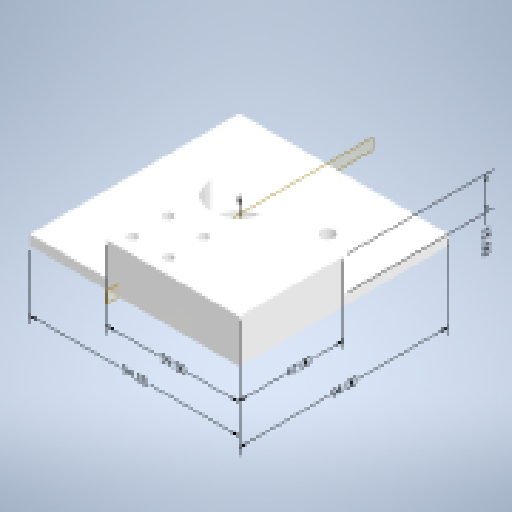
# Autodesk Inventor part: box cover
Saved by Autodesk Inventor 2025.3 (Build 293356000, 356)
## iProperties
Created: 2026-04-05
Part Number: box cover
Material: Wood (Birch)
Document SubType Name: Modeling
Designer: logien
Density: 0.55 g/cm^3
Appearance: Smooth - White
Author: logien
Autodesk Inventor part; units mm, degrees
ref_plane "YZ Plane" through (0, 0, 0) normal (1, 0, 0) x (0, 1, 0)
sketch "Sketch1" plane through (0, 0, 0) normal (0, 1, 0) x (-1, 0, 0)
  line L0 (0, 0) -> (94, 0)
  line L1 (94, 0) -> (94, -94)
  line L2 (94, -94) -> (0, -94)
  line L3 (0, -94) -> (0, 0)
  dimension "d0" = 94
  dimension "d1" = 94
  constraints: 8 end point, 2 parallel, 1 horizontal, 1 perpendicular
  measures "d0" distance of L0.end L1.end
  measures "d1" distance of L0.start L0.end
extrude "Extrusion1" add sketch "Sketch1" along normal blind 4.5
sketch "Sketch2" plane through (0, 4.5, 0) normal (0, 1, 0) x (1, 0, 0)
  circle A0 centre (-47, 47) radius 12.5
  point P0 (0, 0)
  dimension "d4" = 25
  dimension "d5" = 47
  dimension "d6" = 47
  constraints: 1 centre point
  measures "d4" diameter of A0
  measures "d5" horizontal distance of point (0, 0) A0.centre
  measures "d6" horizontal distance of point (0, 0) A0.centre
extrude "Extrusion2" cut sketch "Sketch2" against normal blind 4.5
ref_plane "Work Plane3" through (-54.5, 0, 0) normal (1, 0, 0) x (0, 0, -1)
sketch "Sketch4" plane through (0, 4.5, 0) normal (0, 1, 0) x (1, 0, 0)
  line L0 (0, 94) -> (-94, 94) projected
  line L1 (-94, 94) -> (-94, 0) projected
  line L2 (0, 94) -> (-94, 0)
  circle A0 centre (-27.201, 66.799) radius 3
  line L3 (-94, 94) -> (0, 0)
  circle A1 centre (-66.799, 27.201) radius 3
  circle A2 centre (-55, 23) radius 2
  circle A3 centre (-39, 23) radius 2
  circle A4 centre (-55, 7) radius 2
  circle A5 centre (-39, 7) radius 2
  line L4 (-94, 0) -> (0, 0) projected
  line L5 (-47, 94) -> (-47, 0)
  line L6 (0, 0) -> (0, 94) projected
  circle A6 centre (-47, 47) radius 12.5 projected
  point P0 (-47, 47)
  dimension "d21" = 6
  dimension "d25" = 4
  dimension "d26" = 4
  dimension "d27" = 4
  dimension "d28" = 4
  dimension "d29" = 16
  dimension "d30" = 16
  dimension "d31" = 16
  dimension "d32" = 16
  dimension "d33" = 7
  dimension "d34" = 39
  dimension "d35" = 7
  dimension "d36" = 39
  dimension "d66" = 28
  constraints: 6 centre point, 6 end point, 3 midpoint, 1 point on line, 1 symmetric about line, 1 other
  measures "d21" diameter of A0
  measures "d25" diameter of A2
  measures "d26" diameter of A3
  measures "d27" diameter of A4
  measures "d28" diameter of A5
  measures "d29" distance of A4.centre A2.centre
  measures "d30" distance of A5.centre A3.centre
  measures "d31" distance of A5.centre A4.centre
  measures "d32" distance of A2.centre A3.centre
  measures "d33" distance from line of L4 A4.centre
  measures "d34" distance from line of L1 A4.centre
  measures "d35" distance from line of L4 A5.centre
  measures "d36" distance from line of L6 A3.centre
  measures "d66" distance of A6.centre A0.centre
extrude "Extrusion4" cut sketch "Sketch4" against normal blind 10 contours A0 L2 | L2 A0 | A1 L2 | L2 A1
extrude "Extrusion5" cut sketch "Sketch4" against normal blind 10 contours A2 | A3 | A4 | A5
sketch "Sketch5" plane through (0, 4.5, 0) normal (0, 1, 0) x (1, 0, 0)
  circle A0 centre (-47, 47) radius 12.5 projected
  line L0 (-59.5, 47) -> (-59.5, 0)
  line L1 (-59.5, 47) -> (0, 47)
  line L2 (0, 0) -> (0, 94) projected
  circle A1 centre (-47, 47) radius 12.5
  line L3 (-94, 0) -> (0, 0) projected
  line L4 (-59.5, 0) -> (0, 0)
  line L5 (0, 0) -> (0, 47)
  circle A2 centre (-55, 7) radius 2 projected
  circle A3 centre (-55, 7) radius 2
  circle A4 centre (-55, 23) radius 2 projected
  circle A5 centre (-55, 23) radius 2
  circle A6 centre (-39, 23) radius 2 projected
  circle A7 centre (-39, 23) radius 2
  circle A8 centre (-39, 7) radius 2 projected
  circle A9 centre (-39, 7) radius 2
  point P0 (-34.5, 47)
  constraints: 8 end point, 5 centre point, 5 coincident, 2 vertical, 1 midpoint, 1 perpendicular, 3 other
extrude "Extrusion6" add sketch "Sketch5" along normal blind 15 contours L1 L2 L3 L0 A0
ref_plane "Work Plane5" through (-94, 0, 0) normal (-0.7071, 0, -0.7071) x (0, 1, 0)
ref_plane "Work Plane6" through (0, -10, 0) normal (0, -1, 0) x (1, 0, 0)
body "Solid1"
